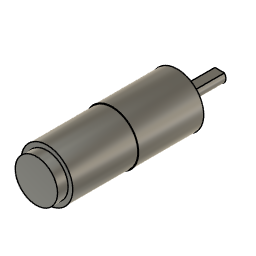
Suspension Partial Axis and Attachment Plate (Autodesk Fusion 360 archive; units mm, degrees)
design "Motor"
Autodesk Fusion 360 part; units mm, degrees
sketch "Sketch1" plane through (0, 0, 0) normal (1, 0, 0) x (0, 1, 0)
  line L0 (0, 7) -> (2, 7)
  line L1 (2, 7) -> (2, 0)
  line L2 (0, 0) -> (0, 12.5)
  line L3 (0, 12.5) -> (-30.8, 12.5)
  line L4 (-30.8, 12.5) -> (-30.8, 0)
  line L5 (-30.8, 12.2) -> (-61.6, 12.2)
  line L6 (-61.6, 12.2) -> (-61.6, 0)
  line L7 (-61.6, 0) -> (0, 0)
  line L8 (2, 3) -> (15, 3)
  line L9 (15, 3) -> (15, 0)
  line L10 (15, 0) -> (0, 0)
  line L11 (-61.6, -12.2) -> (-61.6, 0)
  line L12 (-30.8, -12.2) -> (-61.6, -12.2)
  line L13 (-30.8, -12.5) -> (-30.8, 0)
  line L14 (0, -12.5) -> (-30.8, -12.5)
  line L15 (0, 0) -> (0, -12.5)
  line L16 (0, -7) -> (2, -7)
  line L17 (2, -7) -> (2, 0)
  line L18 (2, -3) -> (15, -3)
  line L19 (15, -3) -> (15, 0)
  dimension "d1" = 25
  dimension "d2" = 24.4
  dimension "d3" = 14
  dimension "d4" = 6
  dimension "d5" = 15
  dimension "d7" = 30.8
  dimension "d8" = 30.8
  dimension "d9" = 2
  constraint horizontal L0
  constraint perpendicular L0 L1
  constraint coincident L2.start L7.end
  constraint vertical L2
  constraint perpendicular L2 L3
  constraint perpendicular L3 L4
  constraint coincident L4 L5.start
  constraint perpendicular L4 L5
  constraint perpendicular L5 L6
  constraint perpendicular L2 L7
  constraint coincident L1 L8.start
  constraint perpendicular L1 L8
  constraint perpendicular L8 L9
  constraint perpendicular L2 L10
  constraint symmetric L0.start L7 L16.start
  constraint symmetric L0.end L7 L16.end
  constraint symmetric L1.end L7 L17.end
  constraint symmetric L2.start L7 L10.end
  constraint symmetric L2.end L7 L14.start
  constraint symmetric L3.end L7 L13.start
  constraint symmetric L4.end L7 L13.end
  constraint symmetric L5.start L7 L12.start
  constraint symmetric L5.end L7 L11.start
  constraint symmetric L6.end L7 L11.end
  constraint symmetric L7 L8.start L18.start
  constraint symmetric L7 L8.end L18.end
  constraint symmetric L7 L9.end L10.start
  constraint coincident L1.end L10
  constraint coincident L0.start L2
  measures "d1" distance of L3 L14
  measures "d2" distance of L5 L12
  measures "d3" distance of L0 L16
  measures "d4" distance of L8 L18
  measures "d5" distance of L2 L19
  measures "d7" distance of L5.start L5.end
  measures "d8" distance of L2.end L3.end
  measures "d9" distance of L0.start L0.end
revolve "Revolve1" add sketch "Sketch1" angle 360 about axis through (0, 1.75, 0) along (0, 1, 0) contours L0 L1 L2 L10 | L2 L3 L4 L7 | L1 L8 L9 L10 | L4 L5 L6 L7
sketch "Sketch2" plane through (0, 15, 0) normal (0, 1, 0) x (-1, 0, 0)
  circle A0 centre (0, 0) radius 3
  circle A1 centre (0, 0) radius 3
  line L0 (-2.2361, 2) -> (2.2361, 2)
  line L1 (0, 0) -> (0, -3)
  point P0 (0, -3)
  dimension "d11" = 6
  dimension "d12" = 5
  constraint concentric A0 A1
  constraint coincident A1 L0.start
  constraint coincident A0 L0.end
  constraint horizontal L0
  constraint coincident A1 P0
  constraint coincident A0.centre A1.centre
  constraint vertical L1
  constraint coincident P0 L1.end
  measures "d11" diameter of A1
  measures "d12" distance of L0 P0
extrude "Extrude1" cut sketch "Sketch2" against normal blind 9 contours A0 A1 L0 picked at (0.5079, 2.7154)
sketch "Sketch3" plane through (0, 0, 0) normal (0, 1, 0) x (-1, 0, 0)
  circle A0 centre (0, 0) radius 12.5
  circle A1 centre (0, 0) radius 7
  circle A2 centre (-6.8943, 6.8943) radius 1.5
  circle A3 centre (6.8943, 6.8943) radius 1.5
  circle A4 centre (6.8943, -6.8943) radius 1.5
  circle A5 centre (-6.8943, -6.8943) radius 1.5
  line L0 (0, 0) -> (-6.8943, 6.8943)
  line L1 (0, 0) -> (6.8943, 6.8943)
  line L2 (6.8943, -6.8943) -> (0, 0)
  line L3 (0, 0) -> (-6.8943, -6.8943)
  circle A6 centre (0, 0) radius 9.75
  line L4 (0, 0) -> (2.2693, 0)
  dimension "d15" = 3
  dimension "d16" = 19.5
  dimension "d20" = 45
  constraint equal A2 A3
  constraint equal A3 A4
  constraint equal A2 A5
  constraint coincident A0.centre A1.centre
  constraint coincident A2.centre L0.end
  constraint coincident A3.centre L1.end
  constraint coincident A4.centre L2.start
  constraint coincident A5.centre L3.end
  constraint perpendicular L2 L3
  constraint perpendicular L1 L2
  constraint perpendicular L0 L1
  constraint concentric A0 A6
  constraint horizontal L4
  constraint coincident A4.centre A6
  constraint coincident A5.centre A6
  constraint coincident A3.centre A6
  constraint coincident A2.centre A6
  measures "d15" diameter of A2
  measures "d16" diameter of A6
  measures "d20" angle of L2 L4
extrude "Extrude2" cut sketch "Sketch3" against normal blind 4.6 contours A3 L1 A6 | A3 L1 A6 | A4 L2 A6 | A4 L2 A6 | A2 L0 A6 | A2 L0 A6 | A3 A6 | A5 L3 A6 | A5 L3 A6 | A4 A6 | A2 A6 | A5 A6
sketch "Sketch4" plane through (0, -61.6, 0) normal (0, -1, 0) x (1, 0, 0)
  circle A0 centre (0, 0) radius 12.2
  circle A1 centre (0, 0) radius 10
  dimension "d23" = 20
  constraint coincident A0.centre A1.centre
  measures "d23" diameter of A1
extrude "Extrude3" add sketch "Sketch4" along normal blind 5 contours A1
extrude "Extrude4" add 1 faces at (-0.8806, 15, 0.6643) along direction (0, 1, 0) blind 5
equation "d16 = 14 mm + ( ( 25 - 14 ) / 2 ) * 1 mm"

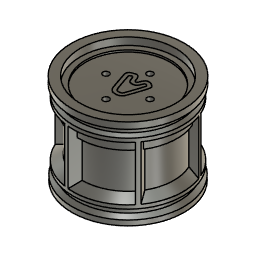
design "Felge"
Autodesk Fusion 360 part; units mm, degrees
sketch "Skizze1" plane through (0, 0, 0) normal (1, 0, 0) x (0, 1, 0)
  line L0 (0, 0) -> (-30.55, 0)
  line L1 (-30.55, 0) -> (-30.55, 2.75)
  line L2 (-30.55, 2.75) -> (-28, 2.75)
  line L3 (-28, 2.75) -> (-28, 7.5)
  line L4 (-28, 7.5) -> (-30, 7.5)
  line L5 (-30, 7.5) -> (-30, 9.5)
  line L6 (-30, 9.5) -> (-25, 9.5)
  line L7 (-25, 9.5) -> (-25, 33)
  line L8 (-25, 33) -> (-26.75, 33)
  line L9 (-26.75, 33) -> (-26.75, 39)
  line L10 (-26.75, 39) -> (-30, 39)
  line L11 (-30, 41) -> (-28, 41)
  line L12 (-28, 41) -> (-28, 45.75)
  line L13 (-28, 45.75) -> (-30.8, 45.75)
  line L14 (-30.8, 45.75) -> (-30.8, 49.25)
  line L15 (-30.8, 49.25) -> (0, 49.25)
  line L16 (0, 49.25) -> (0, 0)
  line L17 (-30, 41) -> (-30, 39)
  line L18 (-23, 49.25) -> (-23, 0)
  line L19 (-23, 41.25) -> (0, 41.25)
  line L20 (-23, 44.25) -> (0, 44.25)
  line L21 (-26, 45.25) -> (-23, 45.25)
  line L22 (-23, 35) -> (-24.75, 35)
  line L23 (-24.75, 35) -> (-24.75, 41)
  line L24 (-24.75, 41) -> (-26, 41)
  line L25 (-26, 41) -> (-26, 49.25)
  line L26 (-23, 7.5) -> (-26, 7.5)
  line L27 (-26, 7.5) -> (-26, 0)
  line L28 (-24.75, 41) -> (-23, 41)
  dimension "d2" = 2.75
  dimension "d3" = 4.75
  dimension "d4" = 2
  dimension "d5" = 23.5
  dimension "d6" = 6
  dimension "d7" = 2
  dimension "d8" = 4.75
  dimension "d9" = 3.5
  dimension "d10" = 49.25
  dimension "d11" = 25
  dimension "d12" = 26.75
  dimension "d16" = 30
  dimension "d17" = 30.8
  dimension "d18" = 28
  dimension "d19" = 28
  dimension "d20" = 30
  dimension "d21" = 30.55
  dimension "d22" = 2
  dimension "d25" = 8
  dimension "d26" = 3
  dimension "d51" = 4
  dimension "d56" = 2
  dimension "d57" = 2
  dimension "d58" = 2
  dimension "d59" = 2
  dimension "d60" = 2
  dimension "d57" = 2
  constraint coincident L0.start L16.end
  constraint horizontal L0
  constraint perpendicular L0 L1
  constraint perpendicular L1 L2
  constraint perpendicular L2 L3
  constraint perpendicular L3 L4
  constraint perpendicular L4 L5
  constraint perpendicular L5 L6
  constraint perpendicular L6 L7
  constraint perpendicular L7 L8
  constraint perpendicular L6 L9
  constraint perpendicular L9 L10
  constraint perpendicular L11 L12
  constraint perpendicular L12 L13
  constraint perpendicular L13 L14
  constraint perpendicular L14 L15
  constraint perpendicular L15 L16
  constraint perpendicular L11 L17
  constraint coincident L15 L18.start
  constraint coincident L0 L18.end
  constraint perpendicular L0 L18
  constraint coincident L18 L19.start
  constraint coincident L16 L19.end
  constraint perpendicular L16 L19
  constraint coincident L18 L20.start
  constraint coincident L16 L20.end
  constraint perpendicular L16 L20
  constraint coincident L18 L21.end
  constraint perpendicular L18 L21
  constraint coincident L18 L22.start
  constraint perpendicular L18 L22
  constraint perpendicular L22 L23
  constraint perpendicular L23 L24
  constraint coincident L15 L25.end
  constraint perpendicular L15 L25
  constraint coincident L18 L26.start
  constraint perpendicular L18 L26
  constraint coincident L0 L27.end
  constraint perpendicular L0 L27
  constraint coincident L18 L28.end
  constraint perpendicular L18 L28
  measures "d2" distance of L0.end L1.end
  measures "d3" distance of L2.end L3.end
  measures "d4" distance of L4.end L5.end
  measures "d5" distance of L6.end L7.end
  measures "d6" distance of L8.end L9.end
  measures "d7" distance of L10.end L11.start
  measures "d8" distance of L11.end L12.end
  measures "d9" distance of L13.end L14.end
  measures "d10" distance of L0 L15
  measures "d11" distance of L7 L16
  measures "d12" distance of L9 L16
  measures "d16" distance of L16 L17
  measures "d17" distance of L14 L16
  measures "d18" distance of L12 L16
  measures "d19" distance of L3 L16
  measures "d20" distance of L5 L16
  measures "d21" distance of L1 L16
  measures "d22" distance of L7 L18
  measures "d25" distance of L15 L19
  measures "d26" distance of L19 L20
  measures "d51" distance of L15 L21
  measures "d56" distance of L3 L27
  measures "d57" distance of L6 L26
  measures "d58" distance of L8 L22
  measures "d59" distance of L9 L23
  measures "d60" distance of L10 L24
  measures "d61" distance of L12 L25
revolve "Drehen2" add sketch "Skizze1" angle 360 about axis through (0, 0, 49.25) along (0, 0, -1) contours L16 L18 L19 L20 | L0 L1 L2 L3 L4 L5 L6 L7 L8 L9 L10 L11 L12 L13 L14 L15 L17 L18 L22 L23 L24 L25 L26 L27 | L18 L21 L24 L25 L28 | L18 L22 L23 L28 makes body 1
sketch "Skizze2" plane through (0, 0, 44.25) normal (0, 0, 1) x (-1, 0, 0)
  circle A0 centre (0, 0) radius 23
  circle A1 centre (0, 0) radius 12
  circle A2 centre (0, -12) radius 1.65
  circle A3 centre (0, 12) radius 1.65
  line L0 (0, 0) -> (0, 12)
  line L1 (0, 0) -> (0, -12)
  line L2 (0, 0) -> (-12, 0)
  line L3 (0, 0) -> (12, 0)
  circle A4 centre (-12, 0) radius 1.65
  circle A5 centre (12, 0) radius 1.65
  dimension "d27" = 24
  dimension "d28" = 3.3
  constraint coincident A0.centre A1.centre
  constraint coincident A1 A2.centre
  constraint coincident A1 A3.centre
  constraint coincident A3.centre L0.end
  constraint coincident A2.centre L1.end
  constraint coincident A1 L2.end
  constraint perpendicular L0 L2
  constraint coincident A1 L3.end
  constraint perpendicular L1 L3
  constraint perpendicular L1 L2
  constraint horizontal L2
  constraint coincident L2.end A4.centre
  constraint coincident L3.end A5.centre
  constraint equal A2 A4
  constraint equal A3 A4
  constraint equal A3 A5
  measures "d27" diameter of A1
  measures "d28" diameter of A2
extrude "Extrusion1" cut sketch "Skizze2" against normal blind 10 contours A1 L3 A5 | A1 A5 | A1 L3 A5 | A1 A3 L0 | A1 A3 | A1 A2 | A1 A2 L1 | A1 A3 L0 | A1 A2 L1 | A1 L2 A4 | A1 L2 A4 | A1 A4 bodies 1
chamfer "Chamfer2" distance 1.15 angle 60 1 edges at (-26.1052, -10.1252, 41) measured on face at (2.7879, -27.8609, 42.5833) on bodies 1
chamfer "Chamfer2" distance 1.47 angle 60 1 edges at (-26.1052, -10.1252, 2.75) measured on face at (1.3957, -27.9652, 4.3333) on bodies 1
chamfer "Chamfer2" distance 2.88 angle 60 1 edges at (-23.3082, -9.0404, 9.5) measured on face at (1.2461, -24.9689, 17.3333) on bodies 1
sketch "Skizze3" plane through (0, 0, 9.5) normal (0, 0, 1) x (-1, 0, 0)
  circle A0 centre (0, 0) radius 30
  circle A1 centre (0, 0) radius 25
  circle A2 centre (0, 0) radius 30
  line L0 (0, 0) -> (0, -25)
  line L1 (0, -25) -> (-2.8106, -29.8681)
  line L2 (-4.958, -29.5875) -> (-2.2508, -24.8985)
  circle A3 centre (0, 0) radius 29.9883
  dimension "d38" = 50
  dimension "d39" = 60
  dimension "d40" = 30
  dimension "d41" = 2
  constraint coincident A0.centre A1.centre
  constraint coincident A1 L0.end
  constraint vertical L0
  constraint coincident A2 L1.end
  constraint coincident A2 L2.start
  constraint coincident A1 L2.end
  constraint parallel L1 L2
  measures "d38" diameter of A1
  measures "d39" diameter of A2
  measures "d40" angle of L0 L1
  measures "d41" distance of L1 L2
extrude "Extrusion2" add sketch "Skizze3" along normal blind 30 contours A0 A2 L1 L2 A3 | A1 L1 L2 A3 picked at (-3.0456, -29.8352) picked at (-2.1855, -26.5701) bodies 1
pattern_circular "C-Anordnung1" count 6 over 360 about axis through (0, 0, 49.25) along (0, 0, -1) of "Extrusion2"
sketch "Skizze4" plane through (0, 0, 44.25) normal (0, 0, 1) x (-1, 0, 0)
  circle A0 centre (0, 12) radius 1.65
  circle A1 centre (12, 0) radius 1.65
  circle A2 centre (-12, 0) radius 1.65
  circle A3 centre (0, -12) radius 1.65
  spline S0 degree 3 poles (-1.422, 6.8614) (-2.0903, 6.6332) (-2.8238, 6.079) (-3.215, 5.5085) knots 0 0 0 0 1 1 1 1
  spline S1 degree 3 poles (-3.215, 5.5085) (-3.8344, 4.6283) (-6.7521, -4.2877) (-6.7684, -5.3798) knots 0 0 0 0 1 1 1 1
  spline S2 degree 3 poles (-6.7684, -5.3798) (-6.7847, -6.1948) (-6.7521, -6.2763) (-6.1164, -6.8631) knots 0 0 0 0 1 1 1 1
  spline S3 degree 3 poles (-6.1164, -6.8631) (-5.6926, -7.2706) (-5.1221, -7.5966) (-4.5516, -7.7596) knots 0 0 0 0 1 1 1 1
  spline S4 degree 3 poles (-4.5516, -7.7596) (-2.889, -8.2323) (-1.8458, -7.6455) (-1.1449, -5.8036) knots 0 0 0 0 1 1 1 1
  spline S5 degree 3 poles (-1.1449, -5.8036) (-0.6722, -4.5648) (-0.5092, -4.2877) (-0.1995, -4.2551) knots 0 0 0 0 1 1 1 1
  spline S6 degree 3 poles (-0.1995, -4.2551) (0.4688, -4.1573) (0.5992, -4.2714) (0.9415, -5.2983) knots 0 0 0 0 1 1 1 1
  spline S7 degree 3 poles (0.9415, -5.2983) (1.3979, -6.6838) (2.0825, -7.7433) (2.7182, -7.9878) knots 0 0 0 0 1 1 1 1
  spline S8 degree 3 poles (2.7182, -7.9878) (3.1583, -8.1834) (3.3539, -8.1508) (4.5437, -7.7433) knots 0 0 0 0 1 1 1 1
  spline S9 degree 3 poles (4.5437, -7.7433) (6.1737, -7.1728) (6.5812, -6.8631) (6.8257, -6.0481) knots 0 0 0 0 1 1 1 1
  spline S10 degree 3 poles (6.8257, -6.0481) (6.9887, -5.5265) (6.9561, -5.2494) (6.6627, -4.2388) knots 0 0 0 0 1 1 1 1
  spline S11 degree 3 poles (6.6627, -4.2388) (6.4671, -3.5705) (6.2389, -2.8859) (6.1574, -2.7066) knots 0 0 0 0 1 1 1 1
  spline S12 degree 3 poles (6.1574, -2.7066) (6.0759, -2.5273) (5.5217, -0.9136) (4.9349, 0.8794) knots 0 0 0 0 1 1 1 1
  spline S13 degree 3 poles (4.9349, 0.8794) (4.3318, 2.6724) (3.7124, 4.4327) (3.5495, 4.7913) knots 0 0 0 0 1 1 1 1
  spline S14 degree 3 poles (3.5495, 4.7913) (3.1746, 5.6063) (2.3596, 6.405) (1.5609, 6.731) knots 0 0 0 0 1 1 1 1
  spline S15 degree 3 poles (1.5609, 6.731) (0.9578, 6.9918) (-0.7863, 7.057) (-1.422, 6.8614) knots 0 0 0 0 1 1 1 1
  spline S16 degree 3 poles (1.3979, 4.5631) (1.7239, 4.2371) (2.2618, 2.868) (3.3702, -0.4246) knots 0 0 0 0 1 1 1 1
  spline S17 degree 3 poles (3.3702, -0.4246) (4.2014, -2.9185) (4.9023, -5.0701) (4.9186, -5.2005) knots 0 0 0 0 1 1 1 1
  spline S18 degree 3 poles (4.9186, -5.2005) (4.9349, -5.4776) (4.0058, -6.0318) (3.5332, -6.0481) knots 0 0 0 0 1 1 1 1
  spline S19 degree 3 poles (3.5332, -6.0481) (3.3539, -6.0481) (3.1257, -5.6569) (2.816, -4.7767) knots 0 0 0 0 1 1 1 1
  spline S20 degree 3 poles (2.816, -4.7767) (2.5552, -4.0921) (2.2455, -3.3586) (2.1314, -3.163) knots 0 0 0 0 1 1 1 1
  spline S21 degree 3 poles (2.1314, -3.163) (1.6098, -2.348) (-0.1669, -2.0383) (-1.2753, -2.5599) knots 0 0 0 0 1 1 1 1
  spline S22 degree 3 poles (-1.2753, -2.5599) (-1.8784, -2.8533) (-2.2859, -3.4401) (-2.726, -4.6626) knots 0 0 0 0 1 1 1 1
  spline S23 degree 3 poles (-2.726, -4.6626) (-2.889, -5.1027) (-3.1498, -5.608) (-3.2965, -5.771) knots 0 0 0 0 1 1 1 1
  spline S24 degree 3 poles (-3.2965, -5.771) (-3.5247, -6.0318) (-3.6225, -6.0318) (-4.193, -5.8362) knots 0 0 0 0 1 1 1 1
  spline S25 degree 3 poles (-4.193, -5.8362) (-4.5516, -5.7058) (-4.8613, -5.4939) (-4.8939, -5.3472) knots 0 0 0 0 1 1 1 1
  spline S26 degree 3 poles (-4.8939, -5.3472) (-4.9428, -5.0701) (-2.1392, 3.4547) (-1.748, 4.2371) knots 0 0 0 0 1 1 1 1
  spline S27 degree 3 poles (-1.748, 4.2371) (-1.4057, 4.8728) (-1.0797, 5.0195) (0.0124, 5.0358) knots 0 0 0 0 1 1 1 1
  spline S28 degree 3 poles (0.0124, 5.0358) (0.86, 5.0358) (1.023, 4.9869) (1.3979, 4.5631) knots 0 0 0 0 1 1 1 1
  circle A4 centre (0, 0) radius 23
extrude "Extrusion3" cut sketch "Skizze4" against normal blind 0.2 contours S0 S1 S2 S3 S4 S5 S6 S7 S8 S9 S10 S11 S12 S13 S14 S15 bodies 1
extrude "Extrusion4" add 1 faces at (-4.8154, 2.7772, 44.05) along direction (0, 0, 1) blind 0.2 separate body on bodies 1 makes body 2
equation "d11 = ( 50 / 2 ) * 1 mm"
equation "d12 = ( 53.5 / 2 ) * 1 mm"
equation "d16 = ( 60 / 2 ) * 1 mm"
equation "d17 = ( 61.6 / 2 ) * 1 mm"
equation "d18 = ( 56 / 2 ) * 1 mm"
equation "d19 = ( 56 / 2 ) * 1 mm"
equation "d20 = ( 60 / 2 ) * 1 mm"
equation "d21 = ( 61.1 / 2 ) * 1 mm"
